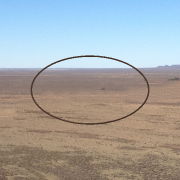
# Autodesk Inventor part: 2h5rbc
Saved by Autodesk Inventor 2013 SP2 (Build 170200200, 200)
## iProperties
Company: HERA Project
Created: 2013-05-20
Part Number: 2h5rbc
Material: Steel, Mild
Document SubType Name: Modeling
Designer: David DeBoer
Density: 7.86 g/cm^3
Description: Hub rebar circle
Mass: 686.463 g
Surface Area: 458.458 cm^2
Volume: 87.3363 cm^3
Author: David DeBoer
Title: Hub rebar
Autodesk Inventor part; units mm, degrees
ref_plane "YZ Plane" through (0, 0, 0) normal (1, 0, 0) x (0, 1, 0)
ref_plane "XZ Plane" through (0, 0, 0) normal (0, 1, 0) x (-1, 0, 0)
ref_plane "XY Plane" through (0, 0, 0) normal (0, 0, 1) x (1, 0, 0)
sketch "Sketch1" plane through (0, 0, 0) normal (0, 0, 1) x (1, 0, 0)
  circle A0 centre (0, 0) radius 3.81
  line L0 (304.8, 3.81) -> (304.8, -3.81) construction
  dimension "d0" = 7.62
  dimension "d1" = 304.8
  constraints: 2 end point, 1 centre point, 1 coincident, 1 vertical
  measures "d0" diameter of A0
  measures "d1" distance from line of L0 point (0, 0)
revolve "Revolution1" add sketch "Sketch1" angle 360 about axis through (304.8, 3.81, 0) along (0, -1, 0)
body "Solid1"
